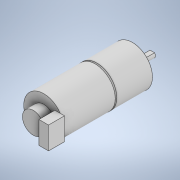
# Autodesk Inventor part: motor
Saved by Autodesk Inventor 2022 (Build 260153000, 153)
## iProperties
Created: 2024-01-09
Part Number: motor
Material: Типовые
Document SubType Name: Modeling
Designer: akapu
Density: 1 g/cm^3
Appearance: По умолчанию
Author: akapu
Autodesk Inventor part; units mm, degrees
ref_plane "YZ Plane" through (0, 0, 0) normal (1, 0, 0) x (0, 1, 0)
ref_plane "XZ Plane" through (0, 0, 0) normal (0, 1, 0) x (-1, 0, 0)
ref_plane "XY Plane" through (0, 0, 0) normal (0, 0, 1) x (1, 0, 0)
sketch "Эскиз1" plane through (0, 0, 0) normal (0, 0, 1) x (1, 0, 0)
  circle A0 centre (0, 0) radius 12.5
  dimension "d0" = 25
  constraints: 1 centre point, 1 coincident
  measures "d0" diameter of A0
extrude "Выдавливание1" add sketch "Эскиз1" along normal blind 55.4
sketch "Эскиз2" plane through (0, 0, 55.4) normal (0, 0, 1) x (1, 0, 0)
  circle A0 centre (0, 0) radius 6.75
  dimension "d3" = 13.5
  constraints: 1 centre point, 1 coincident
  measures "d3" diameter of A0
extrude "Выдавливание2" add sketch "Эскиз2" along normal blind 6.55
sketch "Эскиз3" plane through (0, 0, 55.4) normal (0, 0, 1) x (1, 0, 0)
  line L0 (7, 7) -> (13, 7)
  line L1 (13, 7) -> (13, -7)
  line L2 (13, -7) -> (7, -7)
  line L3 (7, -7) -> (7, 7)
  line L4 (-17.6863, 0) -> (18.6175, 0) projected
  circle A0 centre (0, 0) radius 12.5 projected
  line L5 (-12.5, 0) -> (13, 0)
  point P0 (7, 0)
  dimension "d6" = 6
  dimension "d7" = 14
  dimension "d8" = 25.5
  constraints: 10 end point, 3 point on line, 2 midpoint, 2 parallel, 1 horizontal, 1 horizontal alignment, 1 perpendicular, 1 other
  measures "d6" distance of L1.end L2.end
  measures "d7" distance of L0.end L1.end
  measures "d8" distance of L5.start L5.end
extrude "Выдавливание3" add sketch "Эскиз3" along normal blind 10 contours L0 A0 L4 L3 | L0 L1 L4 A0 | L4 A0 L2 L3 | L4 L1 L2 A0 picked at (8.5105, 3.9415) picked at (8.5105, -3.9415)
sketch "Эскиз4" plane through (0, 0, 0) normal (0, 0, -1) x (-1, 0, 0)
  circle A0 centre (0, 0) radius 3.5
  dimension "d11" = 7
  constraints: 1 centre point, 1 coincident
  measures "d11" diameter of A0
extrude "Выдавливание4" add sketch "Эскиз4" along normal blind 2.7
sketch "Эскиз5" plane through (0, 0, -2.7) normal (0, 0, -1) x (-1, 0, 0)
  circle A0 centre (0, 0) radius 2
  line L0 (1.4283, 1.4) -> (-1.4283, 1.4)
  line L1 (0, -2) -> (0, 1.4)
  dimension "d14" = 4
  dimension "d15" = 3.4
  constraints: 4 end point, 3 point on circle, 1 centre point, 1 coincident, 1 horizontal, 1 midpoint, 1 point on line, 1 vertical
  measures "d14" diameter of A0
  measures "d15" distance of L1.start L1.end
extrude "Выдавливание5" add sketch "Эскиз5" along normal blind 9.7 contours A0 L1 L0 | A0 L0 L1
sketch "Эскиз6" plane through (0, 0, 0) normal (0, 0, -1) x (-1, 0, 0)
  line L0 (0, 8.5) -> (0, -8.5)
  circle A0 centre (0, 8.5) radius 1.5
  circle A1 centre (0, -8.5) radius 1.5
  point P0 (0, 0)
  point P1 (0, 0)
  dimension "d18" = 17
  dimension "d19" = 3
  dimension "d20" = 3
  constraints: 3 coincident, 2 centre point, 2 end point, 1 midpoint, 1 vertical
  measures "d18" distance of L0.start L0.end
  measures "d19" diameter of A0
  measures "d20" diameter of A1
extrude "Выдавливание6" cut sketch "Эскиз6" against normal blind 10
sketch "Эскиз7" plane through (0, 0, 0) normal (0, 1, 0) x (-1, 0, 0)
  line L0 (12.5, 0) -> (-12.5, 0) projected
  line L1 (12.5, 0) -> (12.5, 22.75)
  line L2 (12.5, 0) -> (12.5, 55.4) projected
  circle A0 centre (12.5, 22.75) radius 0.5
  line L3 (-2, -12.4) -> (2, -12.4) projected
  line L4 (0, -12.4) -> (0, 61.95)
  line L5 (6.75, 61.95) -> (-6.75, 61.95) projected
  point P0 (0, 0)
  point P1 (-1.4283, -12.4)
  point P2 (1.4283, -12.4)
  dimension "d23" = 22.75
  dimension "d24" = 1
  constraints: 4 end point, 2 midpoint, 1 centre point, 1 coincident, 1 point on line
  measures "d23" distance of L0.start L1.end
  measures "d24" diameter of A0
revolve "Вращение1" cut sketch "Эскиз7" angle 360 about axis through (0, 0, -12.4) along (0, 0, 1)
